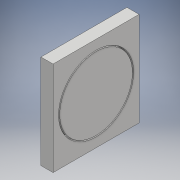
# Autodesk Inventor part: radiator 2018
Saved by Autodesk Inventor 2018.3 (Build 223284000, 284)
## iProperties
Created: 2018-05-19
Part Number: radiator 2018
Material: 一般
Document SubType Name: Modeling
Designer: ku_sk
Density: 1 g/cm^3
Appearance: 既定
Sending System: Autodesk Inventor 2018
Preprocessor: ST-DEVELOPER v17
Title: D:\ku_sk\ドキュメント\Inventor\Aero\KS-15\全体アッセンブリ解析用モデル\body\radiator\radiator 2018.stp
Author: ku_sk
Autodesk Inventor part; units mm, degrees
ref_plane "YZ Plane" through (0, 0, 0) normal (1, 0, 0) x (0, 1, 0)
ref_plane "XZ Plane" through (0, 0, 0) normal (0, 1, 0) x (-1, 0, 0)
ref_plane "XY Plane" through (0, 0, 0) normal (0, 0, 1) x (1, 0, 0)
sketch "スケッチ1" plane through (0, 0, 0) normal (1, 0, 0) x (0, 1, 0)
  line L0 (0, 0) -> (354.9654, 0)
  line L1 (354.9654, 0) -> (354.9654, 388.3801)
  line L2 (354.9654, 388.3801) -> (0, 388.3801)
  line L3 (0, 388.3801) -> (0, 0)
  constraints: 8 end point, 2 parallel, 1 horizontal, 1 perpendicular
extrude "押し出し1" add sketch "スケッチ1" along normal blind 50
sketch "スケッチ2" plane through (50, 0, 0) normal (1, 0, 0) x (0, 0, -1)
  line L0 (-388.3801, 354.9654) -> (-388.3801, 0) projected
  line L1 (-388.3801, 177.4827) -> (0, 177.4827)
  line L2 (0, 0) -> (0, 354.9654) projected
  line L3 (-388.3801, 0) -> (0, 0) projected
  line L4 (-194.19, 0) -> (-194.19, 354.9654)
  line L5 (0, 354.9654) -> (-388.3801, 354.9654) projected
  circle A0 centre (-194.19, 177.4827) radius 150
  circle A1 centre (-194.19, 177.4827) radius 155
  point P0 (-194.19, 177.4827)
  dimension "d2" = 300
  dimension "d3" = 5
  constraints: 5 midpoint, 4 end point, 2 centre point, 1 coincident
  measures "d2" diameter of A0
  measures "d3" radial gap between concentric circles of A0 A1
extrude "押し出し2" cut sketch "スケッチ2" against normal through all contours A1 L4 A0 L1 | L1 A0 L4 A1 | A1 L1 A0 L4 | L4 A0 L1 A1
